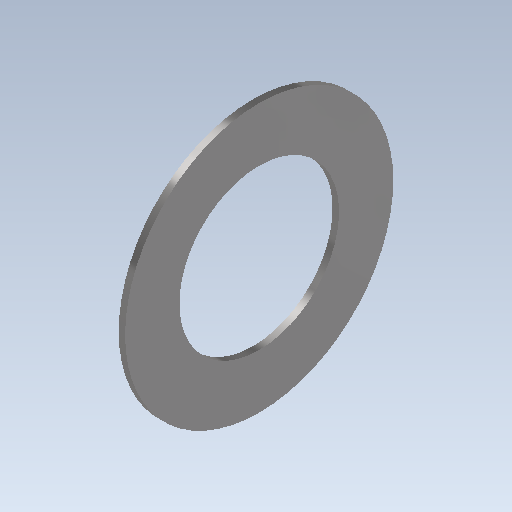
# Autodesk Inventor part: washer_BA2542
Saved by Autodesk Inventor 2020 (Build 240168000, 168)
## iProperties
Created: 2016-05-01
Part Number: washer_BA2542
Catalog Web Link: www.cadenas.de
Description: BA_ _ _ _washer-Thrust Needle Roller Bearings with Retainers
Vendor: MISUMI
Document SubType Name: Modeling
Designer: psAdmin
Manufacturer: MISUMI
Mass: 20 g
Surface Area: 19.9962 cm^2
Volume: 0.894569 cm^3
Density: 22.3571 g/cm^3
Material: ステンレス鋼 440C
Appearance: 半つや出し
Category: PARTsolutions
Company: MISUMI
PSOL_IDENT_0: {$CADENAS_DATA\23d-libs\misumi\metric\12_bearing_holders\washer_ba1024.prj},177 {VTYP=3D},{NB=washer
PSOL_IDENT_1: _BA2542},{LINA=washer_BA2542},{NN=BA_ _ _ _washer},{DATE=21.07.2015 12:46:49},{GEOMDATE=24.05.2010 0
PSOL_IDENT_2: 0:00:00},{VERSION=},{LINEID=60},{LINESUBID=-1},{WBVAR=}  {NB=washer_BA2542},{LINA=washer_BA2542},{KT=
PSOL_IDENT_3: DUMMY},{TYPE=BA2542},{MAT=SUJ2(52100 Bearing Steel)(1.3505_100Cr6) or Equivalent},{DD=25},{DDTOL=+0.
PSOL_IDENT_4: 250/+0.004},{D=42},{DTOL=-0.130/-0.520},{B=2},{BTOL=0/-0.01},{F=41},{F1=29},{DD1=25},{DD1TOL=+0.370/
PSOL_IDENT_5: +0.040},{D1=42},{D1TOL=-0.050/-0.440},{B1=1},{B1TOL=+0.05/-0.05},{MASS=21},{CA=14.7},{COA=58.0}
NN: BA_ _ _ _washer
NT: Thrust Needle Roller Bearings with Retainers
NB: washer_BA2542
NBSYN: washer_$TYPE.
LINA: washer_BA2542
TYPE: BA2542
MAT: SUJ2(52100 Bearing Steel)(1.3505_100Cr6) or Equivalent
DD: 25
DDTOL: +0.250/+0.004
D: 42
DTOL: -0.130/-0.520
B: 2
BTOL: 0/-0.01
F: 41
F1: 29
DD1: 25
DD1TOL: +0.370/+0.040
D1: 42
D1TOL: -0.050/-0.440
B1: 1
B1TOL: +0.05/-0.05
MASS: 21
CA: 14.7
COA: 58.0
SUPPLIER: MISUMI
ARTICLENO: washer_BA2542
BOMINFO: washer_BA2542
CREATOR: CADENAS GmbH
Title: washer_BA2542
Author: Cadenas PARTsolutions
Comments: Thrust Needle Roller Bearings with Retainers
Autodesk Inventor part; units mm, degrees
sketch "Sketch_1" plane through (0, 0, 0) normal (0, 0, 1) x (1, 0, 0)
  line L0 (50, 0) -> (-50, 0)
  line L1 (-0.5, 12.5) -> (0.5, 12.5)
  line L2 (0.5, 12.5) -> (0.5, 21)
  line L3 (0.5, 21) -> (-0.5, 21)
  line L4 (-0.5, 21) -> (-0.5, 12.5)
  constraints: 10 end point
revolve "Revolution1" add sketch "Sketch_1" angle 360 about axis through (50, 0, 0) along (1, 0, 0)
ref_plane "washer1_XY" through (0, 0, 0) normal (1, 0, 0) x (0, 0, -1)
ref_plane "washer1_YZ" through (0, 0, 0) normal (0, 0, -1) x (0, 1, 0)
ref_plane "washer1_ZX" through (0, 0, 0) normal (0, 1, 0) x (1, 0, 0)
ref_plane "washer2_XY" through (0, 0, 0) normal (1, 0, 0) x (0, 0, -1)
ref_plane "washer2_YZ" through (0, 0, 0) normal (0, 0, -1) x (0, 1, 0)
ref_plane "washer2_ZX" through (0, 0, 0) normal (0, 1, 0) x (1, 0, 0)
body "Solid1"
